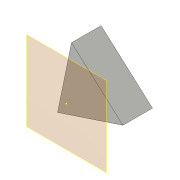
# Autodesk Inventor part: girlNT
Saved by Autodesk Inventor 2016 (Build 200138000, 138)
## iProperties
Created: 2016-01-28
Part Number: girlNT
Material: Generic
Document SubType Name: Modeling
Designer: 301278
Density: 1 g/cm^3
Appearance: Default
Author: 301278
Autodesk Inventor part; units mm, degrees
ref_plane "YZ Plane" through (0, 0, 0) normal (1, 0, 0) x (0, 1, 0)
ref_plane "XZ Plane" through (0, 0, 0) normal (0, 1, 0) x (-1, 0, 0)
ref_plane "XY Plane" through (0, 0, 0) normal (0, 0, 1) x (1, 0, 0)
sketch "Sketch1" plane through (0, 0, 0) normal (0, 0, 1) x (1, 0, 0)
  line L0 (-3.4267, 10.372) -> (10.6957, -2.2184)
  line L1 (10.6957, -2.2184) -> (-7.2691, -8.1536)
  line L2 (-7.2691, -8.1536) -> (-3.4267, 10.372)
  ellipse E0 centre (0, 0) end of major axis (3.175, 0) minor radius 2.667
  dimension "d1" = 3.175
  dimension "d2" = 2.667
  dimension "d0" = 14.1224
  constraints: 6 end point, 2 coincident, 9 other
  measures "d0" horizontal distance of L0.end L0.start
extrude "Extrusion1" add sketch "Sketch1" along normal blind 8.128 contours L0 L1 L2 | E0
ref_plane "Work Plane2" through (0, 0, 12.954) normal (0, 0, 1) x (1, 0, 0)
sketch "Sketch2" plane through (0, 0, 12.954) normal (0, 0, 1) x (1, 0, 0)
  point P0 (0, 0)
sketch "Sketch3" plane through (0, 0, 12.954) normal (0, 0, 1) x (1, 0, 0)
  point P0 (0, 0)
body "Solid1"
